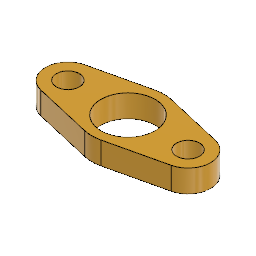
Z_Nut_Retainer v1 (Autodesk Fusion 360 design; units mm, degrees)
Autodesk Fusion 360 part; units mm, degrees
sketch "Sketch1" plane through (0, 0, 0) normal (0, 0, 1) x (1, 0, 0)
  circle A0 centre (-13.3, 0) radius 2.55
  circle A1 centre (-13.3, 0) radius 5
  line L0 (0, 10) -> (0, 0) construction
  circle A2 centre (13.3, 0) radius 2.55
  circle A3 centre (13.3, 0) radius 5
  circle A4 centre (0, 0) radius 6
  circle A5 centre (0, 0) radius 8
  line L1 (-14.2326, 4.9123) -> (-1.8069, 7.7933)
  line L2 (1.8045, 7.7938) -> (14.4278, 4.8711)
  line L3 (1.8045, -7.7938) -> (14.4278, -4.8711)
  line L4 (-14.4278, -4.8711) -> (-1.8045, -7.7938)
  circle A6 centre (-13.3, 0) radius 1.5
  circle A7 centre (13.3, 0) radius 1.5
  dimension "d1" = 5.1
  dimension "d2" = 13.3
  dimension "d3" = 10
  dimension "d6" = 12
  dimension "d7" = 16
  dimension "d10" = 3
  constraint concentric A0 A1
  constraint vertical L0
  constraint coincident L0.end A4.centre
  constraint symmetric A0 L0 A2
  constraint symmetric A1 L0 A3
  constraint concentric A4 A5
  constraint coincident A1 L1.start
  constraint coincident A5 L1.end
  constraint tangent A5 L1
  constraint coincident A5 L2.start
  constraint coincident A3 L2.end
  constraint tangent A3 L2
  constraint coincident A5 L3.start
  constraint tangent A5 L3
  constraint coincident A3 L3.end
  constraint tangent A3 L3
  constraint coincident A1 L4.start
  constraint tangent A1 L4
  constraint coincident A5 L4.end
  constraint tangent A5 L4
  constraint tangent A5 L2
  constraint concentric A1 A6
  constraint symmetric L0 A6 A7
  measures "d1" diameter of A0
  measures "d2" distance of L0.end A0.centre
  measures "d3" diameter of A1
  measures "d6" diameter of A4
  measures "d7" diameter of A5
  measures "d10" diameter of A6
extrude "Extrude2" add sketch "Sketch1" along normal blind 5 contours A1 | A1 A5 L1 L4 | A5 | A3 A5 L2 L3 | A3
equation "d2 = ( 26.6 / 2 ) * 1 mm"
